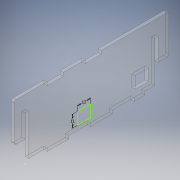
# Autodesk Inventor part: side_v2
Saved by Autodesk Inventor 2017.2 (Build 212233000, 233)
## iProperties
Created: 2017-06-09
Part Number: side_v2
Material: Generic
Document SubType Name: Modeling
Designer: SandeepSH
Density: 1 g/cm^3
Appearance: Polycarbonate - Clear
Author: SandeepSH
Autodesk Inventor part; units mm, degrees
ref_plane "YZ Plane" through (0, 0, 0) normal (1, 0, 0) x (0, 1, 0)
ref_plane "XZ Plane" through (0, 0, 0) normal (0, 1, 0) x (-1, 0, 0)
ref_plane "XY Plane" through (0, 0, 0) normal (0, 0, 1) x (1, 0, 0)
sketch "Sketch1" plane through (0, 0, 0) normal (1, 0, 0) x (0, 1, 0)
  line L0 (0, 0) -> (55.5, 0)
  line L1 (55.5, 0) -> (55.5, -122)
  line L2 (55.5, -122) -> (0, -122)
  line L3 (0, -122) -> (0, 0)
  dimension "d0" = 55.5
  dimension "d1" = 122
  constraints: 8 end point, 2 parallel, 1 horizontal, 1 perpendicular
  measures "d0" distance of L1.end L2.end
  measures "d1" distance of L0.end L1.end
extrude "Extrusion1" add sketch "Sketch1" along normal blind 3
sketch "Sketch2" plane through (3, 0, 0) normal (1, 0, 0) x (0, 0, -1)
  line L0 (0, 0) -> (122, 0) projected
  line L1 (0, 0) -> (20, 0)
  line L2 (20, 0) -> (20, 3)
  line L3 (20, 3) -> (0, 3)
  line L4 (0, 3) -> (0, 0)
  line L5 (40, 0) -> (60, 0)
  line L6 (60, 0) -> (60, 3)
  line L7 (60, 3) -> (40, 3)
  line L8 (40, 3) -> (40, 0)
  line L9 (80, 0) -> (100, 0)
  line L10 (100, 0) -> (100, 3)
  line L11 (100, 3) -> (80, 3)
  line L12 (80, 3) -> (80, 0)
  line L13 (122, 0) -> (120, 0)
  line L14 (120, 0) -> (122, 0)
  line L15 (122, 0) -> (122, 0)
  line L16 (122, 55.5) -> (0, 55.5) projected
  line L17 (20, 55.5) -> (35, 55.5)
  line L18 (35, 55.5) -> (35, 52.5)
  line L19 (35, 52.5) -> (20, 52.5)
  line L20 (20, 52.5) -> (20, 55.5)
  line L21 (0, 55.5) -> (0, 0) projected
  line L22 (55, 55.5) -> (70, 55.5)
  line L23 (70, 55.5) -> (70, 52.5)
  line L24 (70, 52.5) -> (55, 52.5)
  line L25 (55, 52.5) -> (55, 55.5)
  line L26 (0, 3) -> (3, 3)
  line L27 (3, 3) -> (3, 40.5)
  line L28 (3, 40.5) -> (0, 40.5)
  line L29 (0, 40.5) -> (0, 3)
  line L30 (122, 0) -> (119, 0)
  line L31 (119, 0) -> (119, 40.5)
  line L32 (119, 40.5) -> (122, 40.5)
  line L33 (122, 40.5) -> (122, 0)
  line L34 (119, 0) -> (110, 0)
  line L35 (110, 0) -> (110, 3)
  line L36 (110, 3) -> (119, 3)
  line L37 (119, 3) -> (119, 0)
  line L38 (122, 0) -> (122, 55.5) projected
  dimension "d4" = 20
  dimension "d5" = 3
  dimension "d6" = 20
  dimension "d7" = 20
  dimension "d8" = 3
  dimension "d9" = 20
  dimension "d10" = 20
  dimension "d13" = 15
  dimension "d14" = 3
  dimension "d17" = 20
  dimension "d18" = 15
  dimension "d19" = 20
  dimension "d20" = 3
  dimension "d21" = 15
  dimension "d22" = 3
  dimension "d23" = 15
  dimension "d46" = 10
  dimension "d47" = 3
  constraints: 70 end point, 17 equal length, 9 horizontal, 8 perpendicular, 5 point on line, 2 collinear
  measures "d4" distance of L3.end L2.end
  measures "d5" distance of L2.end L1.end
  measures "d6" distance of L7.end L6.end
  measures "d7" distance of L11.end L10.end
  measures "d8" distance of L10.end L9.end
  measures "d9" distance between parallel lines of L8 L2
  measures "d10" distance between parallel lines of L12 L6
  measures "d13" distance of L18.end L19.end
  measures "d14" distance of L17.end L18.end
  measures "d17" distance between parallel lines of L20 L21
  measures "d18" distance of L23.end L24.end
  measures "d19" distance between parallel lines of L25 L18
  measures "d20" distance of L28.end L27.end
  measures "d21" distance between parallel lines of L16 L28
  measures "d22" distance of L31.end L32.end
  measures "d23" distance between parallel lines of L16 L32
  measures "d46" distance between parallel lines of L35 L10
  measures "d47" distance between parallel lines of L0 L36
extrude "Extrusion2" [suppressed]
sketch "Sketch3" plane through (3, 0, 0) normal (1, 0, 0) x (0, 0, -1)
  line L0 (54, 26.1259) -> (54, 15.3243)
  line L1 (0, 55.5) -> (0, 0) projected
  line L2 (0, 55.5) -> (-10, 55.5)
  line L3 (-10, 55.5) -> (-10, 20)
  line L4 (-10, 20) -> (0, 20)
  line L5 (0, 20) -> (0, 55.5)
  line L6 (0, 0) -> (122, 0) projected
  line L7 (119, 3) -> (119, 40.5) projected
  line L8 (122, 55.5) -> (122, 0) projected
  line L9 (122, 55.5) -> (132, 55.5)
  line L10 (132, 55.5) -> (132, 20)
  line L11 (132, 20) -> (122, 20)
  line L12 (122, 20) -> (122, 55.5)
  line L13 (0, 0) -> (122, 0) projected
  point P0 (0, 40.5)
  point P1 (20, 0)
  point P2 (40, 0)
  point P3 (139, 3)
  point P4 (122, 40.5)
  point P5 (100, 0)
  point P6 (120, 0)
  dimension "d26" = 10
  dimension "d27" = 20
  dimension "d28" = 65
  dimension "d29" = 10
  dimension "d30" = 20
  constraints: 18 end point, 4 parallel, 2 horizontal, 2 perpendicular, 1 vertical, 1 other
  measures "d26" distance of L4.end L3.end
  measures "d27" distance between parallel lines of L6 L4
  measures "d29" distance of L10.end L11.end
  measures "d30" distance between parallel lines of L13 L11
extrude "Extrusion3" add sketch "Sketch3" against normal blind 3
fillet "Fillet1" radius 2 4 edges at (1.5, 55.5, 10) (1.5, 20, 10) (1.5, 55.5, -132) (1.5, 20, -132) curvature continuous yes
sketch "Sketch4" plane through (3, 0, 0) normal (1, 0, 0) x (0, 0, -1)
  line L0 (60, 7) -> (48, 7)
  line L1 (48, 7) -> (48, 18)
  line L2 (48, 18) -> (60, 18)
  line L3 (60, 18) -> (60, 7)
  point P0 (0, 0)
  dimension "d34" = 12
  dimension "d35" = 11
  constraints: 8 end point, 2 parallel, 1 horizontal, 1 perpendicular
  measures "d34" distance of L1.end L2.end
  measures "d35" distance of L0.end L1.end
sketch "Sketch5" plane through (3, 0, 0) normal (1, 0, 0) x (0, 0, -1)
  line L0 (101, 9) -> (113, 9)
  line L1 (113, 9) -> (113, 20)
  line L2 (113, 20) -> (101, 20)
  line L3 (101, 20) -> (101, 9)
  line L4 (122, 0) -> (122, 20) projected
  line L5 (0, 0) -> (122, 0) projected
  dimension "d39" = 12
  dimension "d40" = 11
  dimension "d50" = 9
  dimension "d51" = 9
  constraints: 8 end point, 2 parallel, 1 horizontal, 1 perpendicular
  measures "d39" distance of L2.end L1.end
  measures "d40" distance of L1.end L0.end
  measures "d50" distance between parallel lines of L4 L1
  measures "d51" distance between parallel lines of L5 L0
extrude "Extrusion5" cut sketch "Sketch5" against normal through all
extrude "Extrusion6" cut sketch "Sketch2" against normal through all contours L4 L3 L2 L0 | L21 L28 L27 L3 | L8 L7 L6 L0 | L12 L11 L10 L0 | L16 L18 L19 L20 | L35 L36 L31 L0 | L16 L23 L24 L25 | L31 L32 L33 L0
equation "\"d9\" = d4"
equation "\"d10\" = d6"
equation "\"d47\" = d8"
body "Solid1"
